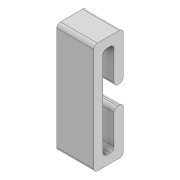
# Autodesk Inventor part: ruziiiii
Saved by Autodesk Inventor 2020 (Build 240168000, 168)
## iProperties
Created: 2025-05-22
Part Number: ruziiiii
Material: Типовые
Document SubType Name: Modeling
Designer: 4s
Density: 1 g/cm^3
Appearance: По умолчанию
Author: 4s
Autodesk Inventor part; units mm, degrees
ref_plane "YZ Plane" through (0, 0, 0) normal (1, 0, 0) x (0, 1, 0)
ref_plane "XZ Plane" through (0, 0, 0) normal (0, 1, 0) x (-1, 0, 0)
ref_plane "XY Plane" through (0, 0, 0) normal (0, 0, 1) x (1, 0, 0)
sketch "Эскиз1" plane through (0, 0, 0) normal (1, 0, 0) x (0, 1, 0)
  line L0 (-1, 0) -> (-24, 0)
  line L1 (-25, -1) -> (-25, -2)
  line L2 (0, -2) -> (0, -1)
  line L3 (1.5, 2.5) -> (-26.5, 2.5)
  line L4 (-27.5, 1.5) -> (-27.5, -4.5)
  line L5 (2.5, -4.5) -> (2.5, 1.5)
  line L6 (-15, -4) -> (-15, -4.5)
  line L7 (-10, -4.5) -> (-10, -4)
  arc A0 (1.5, -5.5) -> (2.5, -4.5) centre (1.5, -4.5) ccw
  arc A1 (2.5, 1.5) -> (1.5, 2.5) centre (1.5, 1.5) ccw
  arc A2 (-26.5, 2.5) -> (-27.5, 1.5) centre (-26.5, 1.5) ccw
  arc A3 (-27.5, -4.5) -> (-26.5, -5.5) centre (-26.5, -4.5) ccw
  arc A4 (-25, -2) -> (-24, -3) centre (-24, -2) ccw
  arc A5 (-24, 0) -> (-25, -1) centre (-24, -1) ccw
  arc A6 (0, -1) -> (-1, 0) centre (-1, -1) ccw
  arc A7 (-1, -3) -> (0, -2) centre (-1, -2) ccw
  line L8 (0.0224, -5.5) -> (-9, -5.5)
  line L9 (-16, -5.5) -> (-16.8462, -5.5)
  line L10 (-24, -3) -> (-16, -3)
  line L11 (-9, -3) -> (-1, -3)
  line L12 (-26.5, -5.5) -> (-15, -5.5)
  line L13 (-10, -5.5) -> (1.5, -5.5)
  arc A8 (-9, -3) -> (-10, -4) centre (-9, -4) ccw
  arc A9 (-10, -4.5) -> (-9, -5.5) centre (-9, -4.5) ccw
  arc A10 (-15, -4) -> (-16, -3) centre (-16, -4) ccw
  arc A11 (-16, -5.5) -> (-15, -4.5) centre (-16, -4.5) ccw
  point P0 (0, 0)
  point P1 (-25, -3)
  point P2 (-25, 0)
  point P3 (0, -3)
  dimension "d0" = 25
  dimension "d1" = 3
  dimension "d4" = 2.5
  dimension "d5" = 2.5
  dimension "d6" = 2.5
  dimension "d7" = 5
  dimension "d8" = 1
  dimension "d9" = 1
  dimension "d10" = 12.5
  dimension "d11" = 1
  dimension "d12" = 1
  constraints: 28 end point, 28 tangent, 24 point on circle, 12 centre point, 11 parallel, 10 point on line, 8 equal radius, 2 horizontal, 2 perpendicular
  measures "d0" distance of point (0, -3) point (-25, -3)
  measures "d1" distance of point (-25, -3) point (-25, 0)
  measures "d4" distance between parallel lines of L0 L3
  measures "d5" distance between parallel lines of L5 L2
  measures "d6" distance between parallel lines of L1 L4
  measures "d7" distance between parallel lines of L6 L7
  measures "d8" radius of A0
  measures "d9" radius of A6
  measures "d10" distance between parallel lines of L5 L7
  measures "d11" radius of A8
  measures "d12" radius of A10
extrude "Выдавливание1" add sketch "Эскиз1" along normal blind 10
